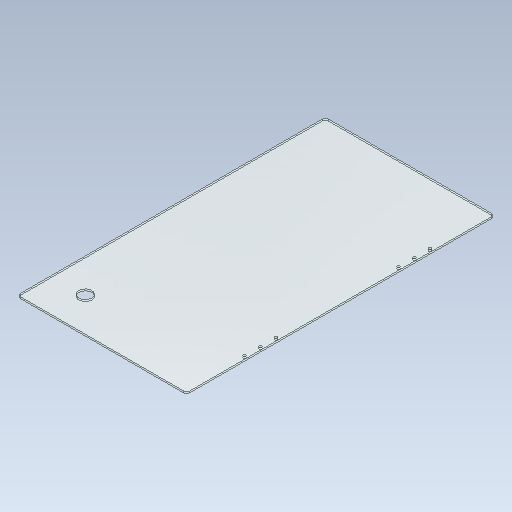
# Autodesk Inventor part: Puerta de Inspección
Saved by Autodesk Inventor 2020 (Build 240168000, 168)
## iProperties
Created: 2020-06-16
Part Number: Puerta de Inspección
Material: Genérico
Document SubType Name: Modeling
Designer: Pipi
Density: 1 g/cm^3
Appearance: Claro
Author: Pipi
Autodesk Inventor part; units mm, degrees
ref_plane "YZ Plane" through (0, 0, 0) normal (1, 0, 0) x (0, 1, 0)
ref_plane "XZ Plane" through (0, 0, 0) normal (0, 1, 0) x (-1, 0, 0)
ref_plane "XY Plane" through (0, 0, 0) normal (0, 0, 1) x (1, 0, 0)
sketch "Boceto1" plane through (0, 0, 0) normal (0, 1, 0) x (-1, 0, 0)
  line L0 (137.798, 30.261) -> (-98.702, 30.261)
  line L1 (-102.702, 26.261) -> (-102.702, -410.739)
  line L2 (-98.702, -414.739) -> (137.798, -414.739)
  line L3 (141.798, -410.739) -> (141.798, 26.261)
  arc A0 (141.798, 26.261) -> (137.798, 30.261) centre (137.798, 26.261) ccw
  arc A1 (-98.702, 30.261) -> (-102.702, 26.261) centre (-98.702, 26.261) ccw
  arc A2 (-102.702, -410.739) -> (-98.702, -414.739) centre (-98.702, -410.739) ccw
  arc A3 (137.798, -414.739) -> (141.798, -410.739) centre (137.798, -410.739) ccw
  line L4 (-102.702, -414.739) -> (-97.452, -414.739)
  circle A4 centre (-97.952, -58.238) radius 2
  circle A5 centre (-97.952, -326.24) radius 2
  circle A6 centre (-97.952, -80.988) radius 2
  circle A7 centre (-97.952, -103.738) radius 2
  circle A8 centre (-97.952, -303.49) radius 2
  circle A9 centre (-97.952, -280.74) radius 2
  circle A10 centre (93.798, -19.739) radius 9.5
  point P0 (141.798, 30.261)
  point P1 (-102.702, 30.261)
  point P2 (141.798, -414.739)
  dimension "d0" = 244.5
  dimension "d1" = 445
  dimension "d2" = 244.5
  dimension "d3" = 4
  dimension "d6" = 5.25
  dimension "d7" = 4
  dimension "d12" = 4
  dimension "d13" = 88.499
  dimension "d14" = 4
  dimension "d15" = 22.75
  dimension "d16" = 4
  dimension "d17" = 22.75
  dimension "d18" = 88.499
  dimension "d19" = 4.75
  dimension "d20" = 4
  dimension "d21" = 22.75
  dimension "d22" = 4.75
  dimension "d23" = 4
  dimension "d24" = 22.75
  dimension "d25" = 4.75
  dimension "d26" = 4.75
  dimension "d27" = 4.75
  dimension "d28" = 4.75
  dimension "d29" = 19
  dimension "d30" = 50
  dimension "d31" = 48
  constraints: 11 centre point, 10 end point, 9 point on line, 8 point on circle, 8 tangent, 3 equal radius, 2 perpendicular, 1 horizontal
  measures "d0" distance of point (141.798, 30.261) point (-102.702, 30.261)
  measures "d1" distance of point (-102.702, 30.261) L4.start
  measures "d2" distance of L4.start point (141.798, -414.739)
  measures "d3" radius of A0
  measures "d6" distance of L4.start L4.end
  measures "d7" diameter of A4
  measures "d12" diameter of A5
  measures "d13" distance from line of L0 A4.centre
  measures "d14" diameter of A6
  measures "d15" distance of A4.centre A6.centre
  measures "d16" diameter of A7
  measures "d17" distance of A6.centre A7.centre
  measures "d18" distance from line of L2 A5.centre
  measures "d19" distance from line of L1 A5.centre
  measures "d20" diameter of A8
  measures "d21" distance of A8.centre A5.centre
  measures "d22" distance from line of L1 A8.centre
  measures "d23" diameter of A9
  measures "d24" distance of A9.centre A8.centre
  measures "d25" distance from line of L1 A9.centre
  measures "d26" distance from line of A7.centre L1
  measures "d27" distance from line of A6.centre L1
  measures "d28" distance from line of A4.centre L1
  measures "d29" diameter of A10
  measures "d30" distance from line of L0 A10.centre
  measures "d31" distance from line of L3 A10.centre
extrude "Extrusión1" add sketch "Boceto1" along normal blind 2.4
equation "\"d0\" = d2"
equation "\"d13\" = d18"
equation "\"d22\" = d19"
equation "\"d25\" = d22"
equation "\"d26\" = d25"
equation "\"d27\" = d26"
equation "\"d28\" = d27"
